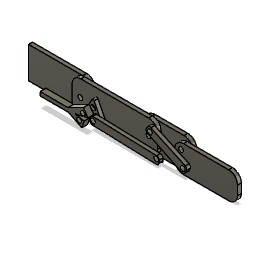
Finger 4 v4 (Autodesk Fusion 360 design; units mm, degrees)
Autodesk Fusion 360 part; units mm, degrees
sketch "Sketch1" plane through (0, 0, 0) normal (0, 0, 1) x (1, 0, 0)
  line L0 (0, 0) -> (50, 0)
  line L1 (50, 0) -> (50, 25)
  line L2 (50, 25) -> (0, 25)
  line L3 (0, 25) -> (0, 0)
  line L4 (90, 0) -> (130, 0)
  line L5 (130, 0) -> (130, 24)
  line L6 (130, 24) -> (90, 24)
  line L7 (90, 24) -> (90, 0)
  dimension "d3" = 50
  dimension "d4" = 40
  dimension "d5" = 25
  dimension "d6" = 24
  dimension "d7" = 40
  constraint horizontal L0
  constraint vertical L1
  constraint horizontal L2
  constraint vertical L3
  constraint coincident L0.start L3.end
  constraint horizontal L4
  constraint vertical L5
  constraint horizontal L6
  constraint vertical L7
  measures "d3" distance of L1.end L2.end
  measures "d4" distance of L5.end L6.end
  measures "d5" distance of L0.start L2.end
  measures "d6" distance of L4.start L6.end
  measures "d7" distance of L1 L7
extrude "Extrude1" add sketch "Sketch1" along normal blind 3 makes body 1 at (16.6667, 16.6667, 0) makes body 2 at (103.3333, 16, 0)
sketch "Sketch2" plane through (0, 0, 3) normal (0, 0, 1) x (1, 0, 0)
  line L0 (0, 25) -> (0, 0)
  line L1 (0, 0) -> (50, 0)
  line L2 (50, 0) -> (50, 25)
  line L3 (50, 25) -> (0, 25)
  line L4 (37.4298, 25) -> (105, 25)
  line L5 (105, 25) -> (105, 0)
  line L6 (105, 0) -> (37.4298, 0)
  line L7 (37.4298, 0) -> (37.4298, 25)
  line L8 (118.586, 21.1734) -> (168.3607, 21.1734)
  line L9 (168.3607, 21.1734) -> (168.3607, 0)
  line L10 (168.3607, 0) -> (118.586, 0)
  line L11 (118.586, 0) -> (118.586, 21.1734)
  constraint horizontal L4
  constraint vertical L5
  constraint horizontal L6
  constraint vertical L7
  constraint coincident L3 L4.start
  constraint horizontal L8
  constraint vertical L9
  constraint horizontal L10
  constraint vertical L11
extrude "Extrude2" add sketch "Sketch2" along normal blind 3 separate body contours L1 L2 L3 L4 L6 L7 | L2 L4 L5 L6 | L8 L9 L10 L11 makes body 3 at (59.9532, 8.3333, 3) makes body 4 at (135.1776, 7.0578, 3)
sketch "Sketch3" plane through (0, 0, 6) normal (0, 0, 1) x (1, 0, 0)
  line L0 (37.4298, 0) -> (105, 0)
  line L1 (105, 0) -> (105, 25)
  line L2 (105, 25) -> (37.4298, 25)
  line L3 (37.4298, 25) -> (37.4298, 0)
  circle A0 centre (123.7043, 16.232) radius 1.85
  line L4 (90, 24) -> (90, 0)
  line L5 (90, 0) -> (130, 0)
  line L6 (130, 0) -> (130, 24)
  line L7 (130, 24) -> (90, 24)
  line L8 (0, 25) -> (0, 0)
  line L9 (0, 0) -> (50, 0)
  line L10 (50, 0) -> (50, 25)
  line L11 (50, 25) -> (0, 25)
  circle A1 centre (97.8747, 12.8837) radius 1.85
  circle A2 centre (44, 12) radius 1.85
  dimension "d10" = 3.7
  dimension "d11" = 3.7
  dimension "d12" = 3.7
  measures "d10" diameter of A0
  measures "d11" diameter of A1
  measures "d12" diameter of A2
extrude "Extrude3" cut sketch "Sketch3" against normal blind 6 contours A0 | A1 | A2 bodies 1 2 3 4
copy_body "Body->Comp1" bodies 1 removing the originals makes body 5 in component "Component"
copy_body "Body->Comp2" bodies 4 removing the originals makes body 6 in component "Component'"
copy_body "Body->Comp3" bodies 2 removing the originals makes body 7 in component "Component''"
copy_body "Body->Comp4" bodies 3 removing the originals makes body 8 in component "Component'''"
sketch "Sketch4" plane through (0, 0, 6) normal (0, 0, 1) x (1, 0, 0)
  circle A0 centre (44, 12) radius 1.85
  circle A1 centre (97.8747, 12.8837) radius 1.85
  line L0 (37.4298, 0) -> (105, 0)
  line L1 (105, 0) -> (105, 25)
  line L2 (105, 25) -> (37.4298, 25)
  line L3 (37.4298, 25) -> (37.4298, 0)
  line L4 (57, 20) -> (49, 4)
  line L5 (49, 4) -> (65, 4)
  line L6 (65, 4) -> (57, 20)
  constraint horizontal L5
extrude "Extrude4" add sketch "Sketch4" along normal blind 3 separate body contours L4 L5 L6 makes body 9
fillet "Fillet1" radius 1 3 edges at (57, 20, 7.5) (49, 4, 7.5) (65, 4, 7.5) on bodies 9
copy_body "Body->Comp5" bodies 9 removing the originals makes body 10 in component "Component''''"
sketch "Sketch5" plane through (0, 0, 9) normal (0, 0, 1) x (1, 0, 0)
  arc A0 (63.382, 4) -> (64.2764, 5.4472) centre (63.382, 5) ccw
  line L0 (64.2764, 5.4472) -> (57.8944, 18.2111)
  arc A1 (57.8944, 18.2111) -> (56.1056, 18.2111) centre (57, 17.7639) ccw
  line L1 (56.1056, 18.2111) -> (49.7236, 5.4472)
  arc A2 (49.7236, 5.4472) -> (50.618, 4) centre (50.618, 5) ccw
  line L2 (50.618, 4) -> (63.382, 4)
  circle A3 centre (54, 7) radius 1.85
  circle A4 centre (57, 13) radius 1.85
  circle A5 centre (60, 7) radius 1.85
  dimension "d31" = 3.7
  dimension "d32" = 3.7
  dimension "d33" = 3.7
  measures "d31" diameter of A3
  measures "d32" diameter of A4
  measures "d33" diameter of A5
extrude "Extrude1'" cut sketch "Sketch5" against normal blind 6 contours A3 bodies 8 in component "Component'''"
extrude "Extrude1''" cut sketch "Sketch5" against normal blind 6 contours A3 bodies 10 in component "Component''''"
extrude "Extrude2'" cut sketch "Sketch5" against normal blind 3 contours A4 | A5 bodies 10 in component "Component''''"
chamfer "Chamfer1" distance 1.3 angle 45 2 edges at (58.2752, 6.331, 6) (55.2752, 12.331, 6) on bodies 10 in component "Component''''"
sketch "Sketch6" plane through (0, 0, 9) normal (0, 0, 1) x (1, 0, 0)
  circle A0 centre (57, 13) radius 1.85
  circle A1 centre (60, 7) radius 1.85
  circle A2 centre (54, 7) radius 1.85
  arc A3 (63.382, 4) -> (64.2764, 5.4472) centre (63.382, 5) ccw
  line L0 (64.2764, 5.4472) -> (57.8944, 18.2111)
  arc A4 (57.8944, 18.2111) -> (56.1056, 18.2111) centre (57, 17.7639) ccw
  line L1 (56.1056, 18.2111) -> (49.7236, 5.4472)
  arc A5 (49.7236, 5.4472) -> (50.618, 4) centre (50.618, 5) ccw
  line L2 (50.618, 4) -> (63.382, 4)
  line L3 (56.5023, 9.4538) -> (-4, 9.4538)
  line L4 (-4, 9.4538) -> (-4, 4)
  line L5 (-4, 4) -> (56.5023, 4)
  line L6 (56.5023, 4) -> (56.5023, 9.4538)
  line L7 (59.285, 15.4301) -> (1, 15.4301)
  line L8 (1, 15.4301) -> (1, 11)
  line L9 (1, 11) -> (59.285, 11)
  line L10 (59.285, 11) -> (59.285, 15.4301)
  circle A6 centre (110, 6) radius 1.85
  line L11 (112.3511, 8.2469) -> (57.6459, 10.0364)
  line L12 (57.6459, 10.0364) -> (57.6459, 4)
  line L13 (57.6459, 4) -> (112.3511, 2.2105)
  line L14 (112.3511, 2.2105) -> (112.3511, 8.2469)
  circle A7 centre (102, 19) radius 1.85
  dimension "d41" = 3.7
  dimension "d42" = 3.7
  constraint horizontal L3
  constraint vertical L4
  constraint horizontal L5
  constraint vertical L6
  constraint horizontal L7
  constraint vertical L8
  constraint horizontal L9
  constraint vertical L10
  constraint coincident L0 L7.start
  constraint coincident L2 L12.end
  constraint perpendicular L2 L12
  constraint parallel L11 L13
  constraint parallel L12 L14
  measures "d41" diameter of A6
  measures "d42" diameter of A7
extrude "Extrude5" add sketch "Sketch6" along normal blind 3 separate body contours A3 L0 L2 L11 L12 | A3 L0 L2 L11 L13 L14 | L1 A5 L2 L3 L5 L6 | L1 L7 L9 L10 | L1 A5 L3 L4 L5 | L1 L7 L8 L9 makes body 11 at (94.117, 4.0021, 9) makes body 12 at (14.7167, 6.8179, 9) makes body 13 at (19.05, 13.1434, 9)
extrude "Extrude2''" cut sketch "Sketch6" against normal blind 6 contours A7 bodies 8 in component "Component'''"
chamfer "Chamfer1'" distance 1.3 angle 45 1 edges at (100.2752, 18.331, 3) on bodies 8 in component "Component'''"
extrude "Extrude1'''" cut sketch "Sketch6" against normal blind 9 contours A6 bodies 7 in component "Component''"
sketch "Sketch7" plane through (0, 0, 6) normal (0, 0, 1) x (1, 0, 0)
  circle A0 centre (123.7043, 16.232) radius 1.85
  line L0 (118.586, 0) -> (168.3607, 0)
  line L1 (168.3607, 0) -> (168.3607, 21.1734)
  line L2 (168.3607, 21.1734) -> (118.586, 21.1734)
  line L3 (118.586, 21.1734) -> (118.586, 0)
  circle A1 centre (128, 7) radius 1.85
  dimension "d50" = 3.7
  measures "d50" diameter of A1
extrude "Extrude1''''" cut sketch "Sketch7" against normal blind 3 contours A1 bodies 6 in component "Component'"
chamfer "Chamfer1''" distance 1.3 angle 45 1 edges at (126.2752, 6.331, 3) on bodies 6 in component "Component'"
fillet "Fillet2" radius 2 6 edges at (57.6459, 10.0364, 10.5) (57.6459, 4, 10.5) (56.5023, 9.4538, 10.5) (56.5023, 4, 10.5) (59.285, 11, 10.5) (59.285, 15.4301, 10.5) on bodies 11 12 13
fillet "Fillet1'" radius 7 1 edges at (50, 25, 1.5) on bodies 5 in component "Component"
fillet "Fillet1''" radius 7 2 edges at (37.4298, 25, 4.5) (105, 25, 4.5) on bodies 8 in component "Component'''"
fillet "Fillet1'''" radius 7 1 edges at (130, 24, 1.5) on bodies 7 in component "Component''"
fillet "Fillet1''''" radius 7 4 edges at (118.586, 21.1734, 4.5) (168.3607, 21.1734, 4.5) (168.3607, 0, 4.5) (118.586, 0, 4.5) on bodies 6 in component "Component'"
fillet "Fillet2'" radius 7 1 edges at (50, 0, 1.5) on bodies 5 in component "Component"
fillet "Fillet2''" radius 7 2 edges at (105, 0, 4.5) (37.4298, 0, 4.5) on bodies 8 in component "Component'''"
fillet "Fillet2'''" radius 7 3 edges at (90, 24, 1.5) (130, 0, 1.5) (90, 0, 1.5) on bodies 7 in component "Component''"
sketch "Sketch8" plane through (0, 0, 6) normal (0, 0, 1) x (1, 0, 0)
  circle A0 centre (102, 19) radius 1.85
  circle A1 centre (54, 7) radius 1.85
  circle A2 centre (44, 12) radius 1.85
  circle A3 centre (97.8747, 12.8837) radius 1.85
  arc A4 (37.4298, 7) -> (44.4298, 0) centre (44.4298, 7) ccw
  line L0 (44.4298, 0) -> (98, 0)
  arc A5 (98, 0) -> (105, 7) centre (98, 7) ccw
  line L1 (105, 7) -> (105, 18)
  arc A6 (105, 18) -> (98, 25) centre (98, 18) ccw
  line L2 (98, 25) -> (44.4298, 25)
  arc A7 (44.4298, 25) -> (37.4298, 18) centre (44.4298, 18) ccw
  line L3 (37.4298, 18) -> (37.4298, 7)
  line L4 (98, 18) -> (129, 3)
  line L5 (129, 3) -> (131.8413, 8.8719)
  line L6 (131.8413, 8.8719) -> (101.0791, 22.9497)
  line L7 (101.0791, 22.9497) -> (98, 18)
  constraint coincident A6.centre L4.start
  constraint perpendicular L4 L5
extrude "Extrude2'''" add sketch "Sketch8" along normal blind 3 separate body contours L1 A6 L4 L6 L7 | L1 A6 L4 L5 L6 makes body 14 in component "Component'"
sketch "Sketch9" plane through (0, 0, 9) normal (0, 0, 1) x (1, 0, 0)
  circle A0 centre (102, 19) radius 1.85
  line L0 (101.0791, 22.9497) -> (98, 18)
  line L1 (98, 18) -> (129, 3)
  line L2 (129, 3) -> (131.8413, 8.8719)
  line L3 (131.8413, 8.8719) -> (101.0791, 22.9497)
  arc A1 (118.586, 7) -> (125.586, 0) centre (125.586, 7) ccw
  line L4 (125.586, 0) -> (161.3607, 0)
  arc A2 (161.3607, 0) -> (168.3607, 7) centre (161.3607, 7) ccw
  line L5 (168.3607, 7) -> (168.3607, 14.1734)
  arc A3 (168.3607, 14.1734) -> (161.3607, 21.1734) centre (161.3607, 14.1734) ccw
  line L6 (161.3607, 21.1734) -> (125.586, 21.1734)
  arc A4 (125.586, 21.1734) -> (118.586, 14.1734) centre (125.586, 14.1734) ccw
  line L7 (118.586, 14.1734) -> (118.586, 7)
  circle A5 centre (128, 7) radius 1.85
  circle A6 centre (123.7043, 16.232) radius 1.85
extrude "Extrude3'" cut sketch "Sketch9" against normal blind 3 contours A5 bodies 14 in component "Component'"
fillet "Fillet2''''" radius 2 4 edges at (101.0791, 22.9497, 7.5) (98, 18, 7.5) (131.8413, 8.8719, 7.5) (129, 3, 7.5) on bodies 14 in component "Component'"
fillet "Fillet3" radius 2 2 edges at (112.3511, 8.2469, 10.5) (112.3511, 2.2105, 10.5) on bodies 11
copy_body "Body->Comp6" bodies 11 removing the originals makes body 15 in component "Component'''''"
copy_body "Body->Comp7" bodies 13 removing the originals makes body 16 in component "Component''''''"
copy_body "Body->Comp8" bodies 12 removing the originals makes body 17 in component "Component'''''''"
copy_body "CutPasteBodies1" bodies 14 removing the originals makes body 18
copy_body "Body->Comp9" bodies 18 removing the originals makes body 19 in component "Component''''''''"
sketch "Sketch10" plane through (0, 0, 3) normal (0, 0, 1) x (1, 0, 0)
  arc A0 (43, 0) -> (50, 7) centre (43, 7) ccw
  line L0 (50, 7) -> (50, 18)
  arc A1 (50, 18) -> (43, 25) centre (43, 18) ccw
  line L1 (43, 25) -> (0, 25)
  line L2 (0, 25) -> (0, 0)
  line L3 (0, 0) -> (43, 0)
  circle A2 centre (44, 12) radius 1.85
  line L4 (-37.5966, 7.4986) -> (-22.5211, 7.4986)
  line L5 (-22.5211, 7.4986) -> (-22.5211, 9.4679)
  line L6 (-22.5211, 9.4679) -> (-37.5966, 9.4679)
  line L7 (-37.5966, 9.4679) -> (-37.5966, 7.4986)
  line L8 (-23.2001, 9.4679) -> (-15.153, 13.5084)
  line L9 (-15.153, 13.5084) -> (-13.1837, 10.6224)
  line L10 (-13.1837, 10.6224) -> (-22.5211, 8.4833)
  line L11 (-22.8946, 7.4986) -> (-16, 4)
  line L12 (-16, 4) -> (-15, 7)
  line L13 (-15, 7) -> (-22.5211, 8.4833)
  constraint horizontal L4
  constraint vertical L5
  constraint horizontal L6
  constraint vertical L7
  constraint coincident L6 L8.start
  constraint midpoint L5 L10.end
  constraint coincident L4 L11.start
extrude "Extrude6" add sketch "Sketch10" along normal blind 3 separate body contours L4 L5 L6 L7 | L4 L5 L11 L12 L13 | L5 L6 L8 L9 L10 makes body 20
move_body "Move1" bodies 20 to x (1, 0, 0) y (0, 1, 0) z (0, 0, 1) at (71.7147, 0.2215, 8)
scale "Scale1" factor 1.52636 about (49.1937, 8.7048, 14) bodies 20
move_body "Move2" bodies 20 to x (1, 0, 0) y (0, 1, 0) z (0, 0, 1) at (-3, 1, 0)
move_face "OffsetFaces1" offset 1 1 faces at (53.8469, 8.1955, 12.4736) on bodies 20
move_face "OffsetFaces2" offset 1 1 faces at (56.4921, 12.0641, 12.4736) on bodies 20
sketch "Sketch11" plane through (0, 0, 14) normal (0, 0, 1) x (1, 0, 0)
  line L0 (45.1571, 11.2077) -> (23.1829, 11.2077)
  line L1 (23.1829, 11.2077) -> (23.1829, 8.2018)
  line L2 (23.1829, 8.2018) -> (45.6236, 8.2018)
  line L3 (45.6236, 8.2018) -> (56.1471, 2.8617)
  line L4 (56.1471, 2.8617) -> (57.9923, 8.3972)
  line L5 (57.9923, 8.3972) -> (50.9911, 9.7779)
  line L6 (50.9911, 9.7779) -> (61.0512, 12.0826)
  line L7 (61.0512, 12.0826) -> (57.4399, 17.375)
  line L8 (57.4399, 17.375) -> (45.1571, 11.2077)
  circle A0 centre (57, 13) radius 1.85
  circle A1 centre (60, 7) radius 1.85
  circle A2 centre (54, 7) radius 1.85
  arc A3 (63.382, 4) -> (64.2764, 5.4472) centre (63.382, 5) ccw
  line L9 (64.2764, 5.4472) -> (57.8944, 18.2111)
  arc A4 (57.8944, 18.2111) -> (56.1056, 18.2111) centre (57, 17.7639) ccw
  line L10 (56.1056, 18.2111) -> (49.7236, 5.4472)
  arc A5 (49.7236, 5.4472) -> (50.618, 4) centre (50.618, 5) ccw
  line L11 (50.618, 4) -> (63.382, 4)
extrude "Extrude7" cut sketch "Sketch11" against normal blind 8 contours L6 A0 | A2 picked at (56.4693, 13.0632) bodies 20
move_body "Move3" bodies 20 to x (1, 0, 0) y (0, 1, 0) z (0, 0, 1) at (0, 0, 3)
copy_body "Body->Comp10" bodies 20 removing the originals makes body 21 in component "Component'''''''''"
component "Component" placed x (1, 0, 0) y (0, 1, 0) z (0, 0, 1) at (0, 0, 0)
component "Component'" placed x (1, 0, 0) y (0, 1, 0) z (0, 0, 1) at (0, 0, 0)
component "Component''" placed x (1, 0, 0) y (0, 1, 0) z (0, 0, 1) at (0, 0, 0)
component "Component'''" placed x (1, 0, 0) y (0, 1, 0) z (0, 0, 1) at (0, 0, 0)
component "Component''''" placed x (1, 0, 0) y (0, 1, 0) z (0, 0, 1) at (0, 0, 0)
component "Component'''''" placed x (1, 0, 0) y (0, 1, 0) z (0, 0, 1) at (0, 0, 0)
component "Component''''''" placed x (1, 0, 0) y (0, 1, 0) z (0, 0, 1) at (0, 0, 0)
component "Component'''''''" placed x (1, 0, 0) y (0, 1, 0) z (0, 0, 1) at (0, 0, 0)
component "Component''''''''" placed x (1, 0, 0) y (0, 1, 0) z (0, 0, 1) at (0, 0, 0)
component "Component'''''''''" placed x (1, 0, 0) y (0, 1, 0) z (0, 0, 1) at (0, 0, 0)
